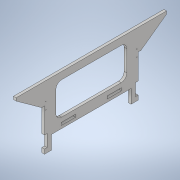
# Autodesk Inventor part: open_case
Saved by Autodesk Inventor 2020 (Build 240168000, 168)
## iProperties
Created: 2019-12-18
Part Number: open_case
Material: Generic
Document SubType Name: Modeling
Designer: fabfarm
Density: 1 g/cm^3
Appearance: Default
Author: fabfarm
Autodesk Inventor part; units mm, degrees
ref_plane "YZ Plane" through (0, 0, 0) normal (1, 0, 0) x (0, 1, 0)
ref_plane "XZ Plane" through (0, 0, 0) normal (0, 1, 0) x (-1, 0, 0)
ref_plane "XY Plane" through (0, 0, 0) normal (0, 0, 1) x (1, 0, 0)
sketch "Sketch1" plane through (0, 0, 0) normal (1, 0, 0) x (0, 1, 0)
  line L0 (-164.075, -330) -> (164.075, -330)
  line L1 (164.075, -330) -> (164.075, 330)
  line L2 (164.075, 330) -> (-164.075, 330)
  line L3 (-164.075, 330) -> (-164.075, -330)
  line L4 (-164.075, -330) -> (164.075, 330) construction
  line L5 (164.075, -330) -> (-164.075, 330) construction
  point P0 (0, 0)
  dimension "d0" = 660
  dimension "d1" = 328.15
  constraints: 12 end point, 2 midpoint, 2 parallel, 1 horizontal, 1 perpendicular
  measures "d0" distance of L0.end L1.end
  measures "d1" distance of L0.start L0.end
extrude "Extrusion1" add sketch "Sketch1" along normal blind 18.55
sketch "Sketch2" plane through (18.55, 0, 0) normal (1, 0, 0) x (0, 0, -1)
  line L0 (-330, 164.075) -> (-330, -164.075) projected
  line L1 (-330, 61.025) -> (-311.45, 61.025)
  line L2 (-311.45, 61.025) -> (-311.45, -39.175)
  line L3 (-311.45, -39.175) -> (-330, -39.175)
  line L4 (-330, -39.175) -> (-330, 61.025)
  line L5 (330, 164.075) -> (-330, 164.075) projected
  line L6 (-330, -164.075) -> (330, -164.075) projected
  point P0 (-330, 163.875)
  point P1 (-330, -163.875)
  point P2 (330, 163.875)
  point P3 (330, -163.875)
  dimension "d20" = 100.2
  dimension "d21" = 103.05
  dimension "d22" = 124.9
  dimension "d23" = 18.55
  constraints: 8 end point, 2 parallel, 1 horizontal, 1 perpendicular, 1 point on line, 2 other
  measures "d20" distance of L1.end L2.end
  measures "d23" distance of L1.start L1.end
extrude "Extrusion2" [suppressed]
mirror "Mirror1" [suppressed]
sketch "Sketch3" plane through (18.55, 0, 0) normal (1, 0, 0) x (0, 0, -1)
  line L0 (210, -114.075) -> (-210, -114.075)
  line L1 (-250, -74.075) -> (-250, 74.075)
  line L2 (-210, 114.075) -> (210, 114.075)
  line L3 (250, 74.075) -> (250, -74.075)
  line L4 (250, -114.075) -> (-250, 114.075) construction
  line L5 (-250, -114.075) -> (250, 114.075) construction
  arc A0 (-210, 114.075) -> (-250, 74.075) centre (-210, 74.075) ccw
  arc A1 (-250, -74.075) -> (-210, -114.075) centre (-210, -74.075) ccw
  arc A2 (250, 74.075) -> (210, 114.075) centre (210, 74.075) ccw
  arc A3 (210, -114.075) -> (250, -74.075) centre (210, -74.075) ccw
  line L6 (-330, 164.075) -> (-330, -164.075) projected
  line L7 (330, 164.075) -> (-330, 164.075) projected
  point P0 (0, 0)
  point P1 (-330, -39.175)
  point P2 (-330, -163.875)
  point P3 (330, 163.875)
  point P4 (-330, 163.875)
  dimension "d17" = 40
  dimension "d40" = 80
  dimension "d41" = 50
  constraints: 12 end point, 8 point on circle, 8 point on line, 8 tangent, 4 centre point, 3 equal radius, 2 midpoint, 2 parallel, 1 horizontal, 1 perpendicular, 1 other
  measures "d17" radius of A0
  measures "d40" distance between parallel lines of L6 L1
extrude "Extrusion3" cut sketch "Sketch3" against normal blind 18.55
sketch "Esquisse4" plane through (18.55, 0, 0) normal (1, 0, 0) x (0, 0, -1)
  circle A0 centre (-312.5725, 59.9025) radius 1.5875
  circle A1 centre (-312.5725, -38.0525) radius 1.5875
  line L0 (-312.5725, 59.9025) -> (-311.45, 61.025) construction
  line L1 (-311.45, 61.025) -> (-311.45, -39.175) projected
  line L2 (210, 114.075) -> (-210, 114.075) projected
  line L3 (0, 114.075) -> (0, -114.075) construction
  line L4 (-210, -114.075) -> (210, -114.075) projected
  circle A2 centre (312.5725, 59.9025) radius 1.5875
  circle A3 centre (312.5725, -38.0525) radius 1.5875
  line L5 (312.5725, 59.9025) -> (311.45, 61.025) construction
  point P0 (0, 0)
  point P1 (311.45, 61.025)
  point P2 (311.45, -39.175)
  point P3 (311.45, -39.175)
  dimension "d24" = 3.175
  dimension "d39" = 45
  constraints: 6 end point, 4 symmetric about line, 2 midpoint, 2 vertical, 1 vertical alignment, 12 other
  measures "d39" angle of L1 L0
extrude "Extrusion4" [suppressed]
sketch "Esquisse5" plane through (18.55, 0, 0) normal (1, 0, 0) x (0, 0, -1)
  line L0 (-211.5, -164.075) -> (-111.4, -164.075)
  line L1 (-111.4, -164.075) -> (-111.4, -145.425)
  line L2 (-111.4, -145.425) -> (-211.5, -145.425)
  line L3 (-211.5, -145.425) -> (-211.5, -164.075)
  line L4 (111.4, -164.075) -> (211.5, -164.075)
  line L5 (211.5, -164.075) -> (211.5, -145.425)
  line L6 (211.5, -145.425) -> (111.4, -145.425)
  line L7 (111.4, -145.425) -> (111.4, -164.075)
  line L8 (-330, 164.075) -> (-330, -164.075) projected
  line L9 (330, -164.075) -> (330, 164.075) projected
  line L10 (210, -114.075) -> (-210, -114.075) projected
  line L11 (-330, -164.075) -> (330, -164.075) projected
  point P0 (0, 0)
  point P1 (-330, -163.875)
  point P2 (330, -163.875)
  point P3 (-330, -39.175)
  point P4 (330, -39.175)
  point P5 (330, 61.025)
  dimension "d27" = 100.1
  dimension "d28" = 100.1
  dimension "d29" = 118.5
  dimension "d30" = 118.5
  dimension "d38" = 18.65
  constraints: 16 end point, 4 parallel, 3 horizontal, 2 perpendicular, 1 collinear, 1 point on line, 1 other
  measures "d27" distance of L1.end L2.end
  measures "d28" distance of L5.end L6.end
  measures "d29" distance between parallel lines of L8 L3
  measures "d30" distance between parallel lines of L9 L5
  measures "d38" distance of L0.end L1.end
extrude "Extrusion5" cut sketch "Esquisse5" against normal blind 20
sketch "Esquisse6" plane through (18.55, 0, 0) normal (1, 0, 0) x (0, 0, -1)
  circle A0 centre (-210.3686, -146.5564) radius 1.6
  circle A1 centre (-112.5314, -146.5564) radius 1.6
  line L0 (-211.5, -164.075) -> (-211.5, -145.425) projected
  line L1 (-211.5, -145.425) -> (-210.3686, -146.5564) construction
  circle A2 centre (112.5314, -146.5564) radius 1.6
  circle A3 centre (210.3686, -146.5564) radius 1.6
  point P0 (0, 0)
  point P1 (-111.4, -145.425)
  point P2 (111.4, -145.425)
  point P3 (211.5, -145.425)
  dimension "d42" = 3.2
  dimension "d43" = 45
  constraints: 3 horizontal alignment, 2 end point, 12 other
  measures "d43" angle of L0 L1
extrude "Extrusion6" cut sketch "Esquisse6" against normal blind 20
sketch "Esquisse8" plane through (18.55, 0, 0) normal (1, 0, 0) x (0, 0, -1)
  line L0 (-330, 164.075) -> (-330, -164.075) projected
  line L1 (-330, -163.875) -> (330, -163.875)
  line L2 (330, -163.875) -> (330, -181.7314)
  line L3 (280, -183.875) -> (-280, -183.875)
  line L4 (-330, -183.875) -> (-330, -163.875)
  line L5 (330, -164.075) -> (330, 164.075) projected
  line L6 (-280, -183.875) -> (-280, -280.325)
  line L7 (-280, -280.325) -> (-330, -280.325)
  line L8 (-330, -280.325) -> (-330, -183.875)
  line L9 (280, -183.875) -> (280, -280.325)
  line L10 (280, -280.325) -> (330, -280.325)
  line L11 (330, -280.325) -> (330, -181.7314)
  point P0 (0, 0)
  point P1 (-330, -39.175)
  point P2 (330, -163.875)
  point P3 (330, -39.175)
  point P4 (330, 61.025)
  dimension "d45" = 20
  dimension "d46" = 116.45
  dimension "d47" = 50
  constraints: 20 end point, 4 parallel, 3 collinear, 2 vertical, 1 horizontal, 1 perpendicular, 1 point on line
  measures "d45" distance between parallel lines of L1 L3
  measures "d46" distance between parallel lines of L7 L1
  measures "d47" distance of L6.end L7.end
extrude "Extrusion7" add sketch "Esquisse8" against normal blind 18.55
sketch "Esquisse9" plane through (18.55, 0, 0) normal (1, 0, 0) x (0, 0, -1)
  line L0 (-330, -248.875) -> (-311.35, -248.875)
  line L1 (-311.35, -248.875) -> (-311.35, -163.675)
  line L2 (-311.35, -163.675) -> (-330, -163.675)
  line L3 (-330, -163.675) -> (-330, -248.875)
  line L4 (330, -248.875) -> (311.35, -248.875)
  line L5 (311.35, -248.875) -> (311.35, -163.675)
  line L6 (311.35, -163.675) -> (330, -163.675)
  line L7 (330, -163.675) -> (330, -248.875)
  line L8 (330, -280.325) -> (330, 164.075) projected
  line L9 (-330, 164.075) -> (-330, -280.325) projected
  line L10 (-330, -280.325) -> (-280, -280.325) projected
  point P0 (0, 0)
  point P1 (330, -39.175)
  point P2 (-330, -39.175)
  dimension "d50" = 85.2
  dimension "d51" = 31.45
  dimension "d52" = 18.65
  constraints: 16 end point, 5 collinear, 4 parallel, 2 horizontal, 2 perpendicular
  measures "d50" distance of L4.end L5.end
  measures "d51" distance between parallel lines of L10 L0
  measures "d52" distance of L0.start L0.end
extrude "Extrusion8" cut sketch "Esquisse9" against normal blind 18.55
sketch "Esquisse10" plane through (18.55, 0, 0) normal (1, 0, 0) x (0, 0, -1)
  line L0 (-330, 14.075) -> (-350, 14.075)
  line L1 (-530, 164.075) -> (-330, 164.075)
  line L2 (-530, 164.075) -> (-530, 144.075)
  line L3 (-530, 144.075) -> (-350, 14.075)
  line L4 (330, 164.075) -> (-330, 164.075) projected
  line L5 (0, 164.075) -> (0, -183.875) construction
  line L6 (-280, -183.875) -> (280, -183.875) projected
  line L7 (-330, 164.075) -> (-330, 14.075)
  line L8 (-330, 164.075) -> (-330, -163.675) projected
  line L9 (330, 14.075) -> (350, 14.075)
  line L10 (530, 164.075) -> (329.9999, 164.075)
  line L11 (530, 164.075) -> (530, 144.075)
  line L12 (530, 144.075) -> (350, 14.075)
  line L13 (329.9999, 164.075) -> (330, 14.075)
  point P0 (0, 0)
  dimension "d56" = 20
  dimension "d59" = 200
  dimension "d67" = 150
  dimension "d68" = 20
  constraints: 22 end point, 4 symmetric about line, 3 collinear, 2 midpoint, 1 horizontal, 1 parallel, 1 vertical
  measures "d56" distance of L1.start L2.end
  measures "d59" distance of L1.start L1.end
  measures "d67" distance of L1.end L0.start
  measures "d68" distance of L0.start L0.end
extrude "Extrusion9" add sketch "Esquisse10" against normal blind 18.55
sketch "Esquisse11" plane through (18.55, 0, 0) normal (1, 0, 0) x (0, 0, -1)
  line L0 (-330, 61.025) -> (-311.45, 61.025) projected
  line L1 (-320.725, 61.025) -> (-320.725, -39.175) construction
  line L2 (-311.45, -39.175) -> (-330, -39.175) projected
  circle A0 centre (-320.725, 36.025) radius 2.25
  circle A1 centre (-320.725, -13.975) radius 2.25
  line L3 (330, 164.075) -> (-330, 164.075) projected
  line L4 (0, 164.075) -> (0, -183.875) construction
  line L5 (-280, -183.875) -> (280, -183.875) projected
  line L6 (330, 61.025) -> (311.45, 61.025)
  line L7 (320.725, 61.025) -> (320.725, -39.175) construction
  line L8 (311.45, -39.175) -> (330, -39.175)
  circle A2 centre (320.725, 36.025) radius 2.25
  circle A3 centre (320.725, -13.975) radius 2.25
  point P0 (0, 0)
  dimension "d62" = 50
  dimension "d63" = 25
  dimension "d64" = 4.5
  constraints: 10 end point, 8 symmetric about line, 4 centre point, 4 midpoint, 4 point on line, 1 equal radius, 2 other
  measures "d62" distance of A1.centre A0.centre
  measures "d63" distance from line of L0 A0.centre
  measures "d64" diameter of A0
extrude "Extrusion10" cut sketch "Esquisse11" against normal blind 18.55
body "Solid1"
